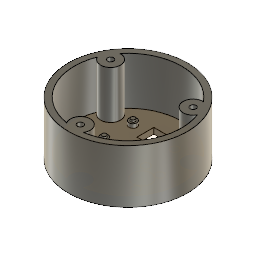
Module (Autodesk Fusion 360 design; units mm, degrees)
Autodesk Fusion 360 part; units mm, degrees
note: some values were not read from the file. Set by a fixed rule: which sketch regions a step uses.
sketch "Sketch1" plane through (0, 0, 0) normal (0, 0, 1) x (1, 0, 0)
  circle A0 centre (0, 0) radius 30
  dimension "d1" = 60
  measures "d1" diameter of A0
extrude "Extrude1" add sketch "Sketch1" along normal blind 27
sketch "Sketch2" plane through (0, 0, 0) normal (0, 0, -1) x (1, 0, 0)
  circle A0 centre (0, 0) radius 30
  line L0 (0, 24) -> (-20.7846, 12)
  line L1 (-20.7846, 12) -> (-20.7846, -12)
  line L2 (-20.7846, -12) -> (0, -24)
  line L3 (0, -24) -> (20.7846, -12)
  line L4 (20.7846, -12) -> (20.7846, 12)
  line L5 (20.7846, 12) -> (0, 24)
  circle A1 centre (0, 24) radius 1.5
  circle A2 centre (20.7846, -12) radius 1.5
  circle A3 centre (-20.7846, -12) radius 1.5
  dimension "d4" = 3
  dimension "d5" = 3
  dimension "d6" = 3
  measures "d4" diameter of A1
  measures "d5" diameter of A2
  measures "d6" diameter of A3
extrude "Extrude2" cut sketch "Sketch2" against normal blind 30 contours L0 L5 A1 | L0 L5 A1 | L1 L2 A3 | L1 L2 A3 | L3 L4 A2 | L3 L4 A2
sketch "Sketch3" plane through (0, 0, 0) normal (0, 0, -1) x (1, 0, 0)
  circle A0 centre (0, 24) radius 1.5
  circle A1 centre (20.7846, -12) radius 1.5
  circle A2 centre (-20.7846, -12) radius 1.5
  circle A3 centre (0, 0) radius 30
  line L0 (2.25, 25.299) -> (0, 26.5981)
  line L1 (0, 26.5981) -> (-2.25, 25.299)
  line L2 (-2.25, 25.299) -> (-2.25, 22.701)
  line L3 (-2.25, 22.701) -> (0, 21.4019)
  line L4 (0, 21.4019) -> (2.25, 22.701)
  line L5 (2.25, 22.701) -> (2.25, 25.299)
  line L6 (23.0821, -10.7869) -> (20.8828, -9.4038)
  line L7 (20.8828, -9.4038) -> (18.5853, -10.6169)
  line L8 (18.5853, -10.6169) -> (18.4871, -13.2131)
  line L9 (18.4871, -13.2131) -> (20.6864, -14.5962)
  line L10 (20.6864, -14.5962) -> (22.9839, -13.3831)
  line L11 (22.9839, -13.3831) -> (23.0821, -10.7869)
  line L12 (-18.5346, -10.701) -> (-20.7846, -9.4019)
  line L13 (-20.7846, -9.4019) -> (-23.0346, -10.701)
  line L14 (-23.0346, -10.701) -> (-23.0346, -13.299)
  line L15 (-23.0346, -13.299) -> (-20.7846, -14.5981)
  line L16 (-20.7846, -14.5981) -> (-18.5346, -13.299)
  line L17 (-18.5346, -13.299) -> (-18.5346, -10.701)
  dimension "d9" = 2.25
  dimension "d10" = 2.25
  dimension "d11" = 2.25
  measures "d9" distance of A3.centre L5
  measures "d10" distance of L11
  measures "d11" distance of L17
extrude "Extrude3" cut sketch "Sketch3" against normal blind 2.4 contours L0 L1 L2 L3 L4 L5 | L6 L7 L8 L9 L10 L11 | L12 L13 L14 L15 L16 L17
sketch "Sketch5" plane through (0, 0, 27) normal (0, 0, 1) x (-1, 0, 0)
  circle A0 centre (0, 24) radius 1.5
  circle A1 centre (-20.7846, -12) radius 1.5
  circle A2 centre (20.7846, -12) radius 1.5
  circle A3 centre (0, 0) radius 30
  circle A4 centre (0, 0) radius 27
  circle A5 centre (0, 24) radius 5
  circle A6 centre (-20.7846, -12) radius 5
  circle A7 centre (20.7846, -12) radius 5
  dimension "d14" = 10
  dimension "d15" = 10
  dimension "d16" = 10
  measures "d14" diameter of A5
  measures "d15" diameter of A6
  measures "d16" diameter of A7
extrude "Extrude4" cut sketch "Sketch5" against normal blind 24 contours A4 A5 A6 A7
sketch "Sketch7" plane through (0, 0, 3) normal (0, 0, 1) x (-1, 0, 0)
  arc A0 (-4.2295, 26.6667) -> (-25.2088, -9.6705) centre (0, 0) ccw
  arc A1 (-20.9792, -16.9962) -> (-25.2088, -9.6705) centre (-20.7846, -12) ccw
  arc A2 (-20.9792, -16.9962) -> (20.9792, -16.9962) centre (0, 0) ccw
  arc A3 (25.2088, -9.6705) -> (20.9792, -16.9962) centre (20.7846, -12) ccw
  arc A4 (25.2088, -9.6705) -> (4.2295, 26.6667) centre (0, 0) ccw
  arc A5 (-4.2295, 26.6667) -> (4.2295, 26.6667) centre (0, 24) ccw
  line L0 (-4.25, -8.75) -> (4.25, -8.75)
  line L1 (4.25, -8.75) -> (4.25, -17.25)
  line L2 (4.25, -17.25) -> (-4.25, -17.25)
  line L3 (-4.25, -17.25) -> (-4.25, -8.75)
  line L4 (-4.25, -8.75) -> (4.25, -17.25) construction
  line L5 (4.25, -8.75) -> (-4.25, -17.25) construction
  dimension "d22" = 8.5
  dimension "d23" = 8.5
extrude "Extrude5" cut sketch "Sketch7" against normal blind 5 contours L0 L1 L2 L3
sketch "Sketch8" plane through (0, 0, 3) normal (0, 0, 1) x (-1, 0, 0)
  line L0 (4.25, -8.75) -> (4.25, -17.25)
  line L1 (4.25, -17.25) -> (-4.25, -17.25)
  line L2 (-4.25, -17.25) -> (-4.25, -8.75)
  line L3 (-4.25, -8.75) -> (4.25, -8.75)
  arc A0 (-4.2295, 26.6667) -> (-25.2088, -9.6705) centre (0, 0) ccw
  arc A1 (-20.9792, -16.9962) -> (-25.2088, -9.6705) centre (-20.7846, -12) ccw
  arc A2 (-20.9792, -16.9962) -> (20.9792, -16.9962) centre (0, 0) ccw
  arc A3 (25.2088, -9.6705) -> (20.9792, -16.9962) centre (20.7846, -12) ccw
  arc A4 (25.2088, -9.6705) -> (4.2295, 26.6667) centre (0, 0) ccw
  arc A5 (-4.2295, 26.6667) -> (4.2295, 26.6667) centre (0, 24) ccw
  line L4 (5, -5) -> (8, -5)
  line L5 (8, -5) -> (8, -21)
  line L6 (8, -21) -> (5, -21)
  line L7 (5, -21) -> (5, -5)
  line L8 (5, -21) -> (-5, -21)
  line L9 (-5, -21) -> (-5, -18)
  line L10 (-5, -18) -> (5, -18)
  line L11 (5, -18) -> (5, -21)
  line L12 (-5, -21) -> (-8, -21)
  line L13 (-8, -21) -> (-8, -5)
  line L14 (-8, -5) -> (-5, -5)
  line L15 (-5, -5) -> (-5, -21)
sketch "Sketch9" plane through (0, 0, 3) normal (0, 0, 1) x (-1, 0, 0)
  line L0 (4.25, -8.75) -> (4.25, -17.25)
  line L1 (4.25, -17.25) -> (-4.25, -17.25)
  line L2 (-4.25, -17.25) -> (-4.25, -8.75)
  line L3 (-4.25, -8.75) -> (4.25, -8.75)
  arc A0 (-4.2295, 26.6667) -> (-25.2088, -9.6705) centre (0, 0) ccw
  arc A1 (-20.9792, -16.9962) -> (-25.2088, -9.6705) centre (-20.7846, -12) ccw
  arc A2 (-20.9792, -16.9962) -> (20.9792, -16.9962) centre (0, 0) ccw
  arc A3 (25.2088, -9.6705) -> (20.9792, -16.9962) centre (20.7846, -12) ccw
  arc A4 (25.2088, -9.6705) -> (4.2295, 26.6667) centre (0, 0) ccw
  arc A5 (-4.2295, 26.6667) -> (4.2295, 26.6667) centre (0, 24) ccw
  circle A6 centre (-15, 8) radius 4.7
  dimension "d28" = 9.4
  measures "d28" diameter of A6
extrude "Extrude7" cut sketch "Sketch9" against normal blind 5 contours A6
sketch "Sketch10" plane through (0, 0, 3) normal (0, 0, 1) x (-1, 0, 0)
  circle A0 centre (-15, 8) radius 4.7
  line L0 (4.25, -8.75) -> (4.25, -17.25)
  line L1 (4.25, -17.25) -> (-4.25, -17.25)
  line L2 (-4.25, -17.25) -> (-4.25, -8.75)
  line L3 (-4.25, -8.75) -> (4.25, -8.75)
  arc A1 (-4.2295, 26.6667) -> (-25.2088, -9.6705) centre (0, 0) ccw
  arc A2 (-20.9792, -16.9962) -> (-25.2088, -9.6705) centre (-20.7846, -12) ccw
  arc A3 (-20.9792, -16.9962) -> (20.9792, -16.9962) centre (0, 0) ccw
  arc A4 (25.2088, -9.6705) -> (20.9792, -16.9962) centre (20.7846, -12) ccw
  arc A5 (25.2088, -9.6705) -> (4.2295, 26.6667) centre (0, 0) ccw
  arc A6 (-4.2295, 26.6667) -> (4.2295, 26.6667) centre (0, 24) ccw
  circle A7 centre (-18, 14) radius 2
  circle A8 centre (-18, 2) radius 2
  dimension "d31" = 4
  dimension "d32" = 4
  measures "d31" diameter of A7
  measures "d32" diameter of A8
extrude "Extrude8" add sketch "Sketch10" along normal blind 11.5 contours A7 | A8
sketch "Sketch13" plane through (0, 0, 3) normal (0, 0, 1) x (-1, 0, 0)
  circle A0 centre (-18, 14) radius 2
  circle A1 centre (-18, 2) radius 2
  circle A2 centre (-15, 8) radius 4.7
  line L0 (4.25, -8.75) -> (4.25, -17.25)
  line L1 (4.25, -17.25) -> (-4.25, -17.25)
  line L2 (-4.25, -17.25) -> (-4.25, -8.75)
  line L3 (-4.25, -8.75) -> (4.25, -8.75)
  arc A3 (-4.2295, 26.6667) -> (-25.2088, -9.6705) centre (0, 0) ccw
  arc A4 (-20.9792, -16.9962) -> (-25.2088, -9.6705) centre (-20.7846, -12) ccw
  arc A5 (-20.9792, -16.9962) -> (20.9792, -16.9962) centre (0, 0) ccw
  arc A6 (25.2088, -9.6705) -> (20.9792, -16.9962) centre (20.7846, -12) ccw
  arc A7 (25.2088, -9.6705) -> (4.2295, 26.6667) centre (0, 0) ccw
  arc A8 (-4.2295, 26.6667) -> (4.2295, 26.6667) centre (0, 24) ccw
  line L4 (0, -13) -> (-10.5, -13)
  line L5 (-10.5, -13) -> (-10.5, 1.5)
  line L6 (-10.5, 1.5) -> (0, 1.5)
  line L7 (0, 1.5) -> (0, -13)
  line L8 (0, -13) -> (10.5, -13)
  line L9 (10.5, -13) -> (10.5, 1.5)
  line L10 (10.5, 1.5) -> (0, 1.5)
  line L11 (0, 1.5) -> (0, -13)
  circle A9 centre (10.5, 1.5) radius 2
  circle A10 centre (-10.5, 1.5) radius 2
  circle A11 centre (10.5, -13) radius 2
  circle A12 centre (-10.5, -13) radius 2
  dimension "d35" = 14.5
  dimension "d36" = 10.5
  dimension "d37" = 14.5
  dimension "d38" = 4
  dimension "d39" = 4
  dimension "d40" = 4
  dimension "d41" = 4
  measures "d38" diameter of A9
  measures "d39" diameter of A10
  measures "d40" diameter of A11
  measures "d41" diameter of A12
extrude "Extrude9" add sketch "Sketch13" along normal blind 2 contours L8 L9 A11 | L8 L9 A11 | L5 L6 A10 | L5 L6 A10 | L9 L10 A9 | L9 L10 A9 | L4 L5 A12 | L4 L5 A12
sketch "Sketch14" plane through (0, 0, 5) normal (0, 0, 1) x (-1, 0, 0)
  circle A0 centre (10.5, -13) radius 2
  circle A1 centre (10.5, -13) radius 1.1
  circle A2 centre (-10.5, -13) radius 1.1
  circle A3 centre (10.5, 1.5) radius 1.1
  circle A4 centre (-10.5, 1.5) radius 1.1
  dimension "d44" = 2.2
  dimension "d45" = 2.2
  dimension "d46" = 2.2
  dimension "d47" = 2.2
  measures "d44" diameter of A1
  measures "d45" diameter of A2
  measures "d46" diameter of A3
  measures "d47" diameter of A4
extrude "Extrude10" add sketch "Sketch14" along normal blind 1 contours A1 | A2 | A3 | A4
sketch "Sketch15" plane through (0, 0, 14.5) normal (0, 0, 1) x (-1, 0, 0)
  circle A0 centre (-18, 2) radius 2
  circle A1 centre (-18, 2) radius 1.1
  circle A2 centre (-18, 14) radius 1.1
  dimension "d50" = 2.2
  dimension "d51" = 2.2
  measures "d50" diameter of A1
  measures "d51" diameter of A2
extrude "Extrude11" add sketch "Sketch15" along normal blind 1 contours A1 | A2
sketch "Sketch16" plane through (0, 0, 3) normal (0, 0, 1) x (-1, 0, 0)
  circle A0 centre (-10.5, -13) radius 2
  circle A1 centre (10.5, -13) radius 2
  circle A2 centre (-10.5, 1.5) radius 2
  circle A3 centre (10.5, 1.5) radius 2
  circle A4 centre (-18, 14) radius 2
  circle A5 centre (-18, 2) radius 2
  circle A6 centre (-15, 8) radius 4.7
  line L0 (4.25, -8.75) -> (4.25, -17.25)
  line L1 (4.25, -17.25) -> (-4.25, -17.25)
  line L2 (-4.25, -17.25) -> (-4.25, -8.75)
  line L3 (-4.25, -8.75) -> (4.25, -8.75)
  arc A7 (-4.2295, 26.6667) -> (-25.2088, -9.6705) centre (0, 0) ccw
  arc A8 (-20.9792, -16.9962) -> (-25.2088, -9.6705) centre (-20.7846, -12) ccw
  arc A9 (-20.9792, -16.9962) -> (20.9792, -16.9962) centre (0, 0) ccw
  arc A10 (25.2088, -9.6705) -> (20.9792, -16.9962) centre (20.7846, -12) ccw
  arc A11 (25.2088, -9.6705) -> (4.2295, 26.6667) centre (0, 0) ccw
  arc A12 (-4.2295, 26.6667) -> (4.2295, 26.6667) centre (0, 24) ccw
sketch "Sketch12" plane through (0, 0, 3) normal (0, 0, 1) x (-1, 0, 0)
  circle A0 centre (-18, 11) radius 2
  circle A1 centre (-18, -1) radius 2
  circle A2 centre (-15, 5) radius 4.7
  line L0 (4.25, -8.75) -> (4.25, -17.25)
  line L1 (4.25, -17.25) -> (-4.25, -17.25)
  line L2 (-4.25, -17.25) -> (-4.25, -8.75)
  line L3 (-4.25, -8.75) -> (4.25, -8.75)
  arc A3 (-4.2295, 26.6667) -> (-25.2088, -9.6705) centre (0, 0) ccw
  arc A4 (-20.9792, -16.9962) -> (-25.2088, -9.6705) centre (-20.7846, -12) ccw
  arc A5 (-20.9792, -16.9962) -> (20.9792, -16.9962) centre (0, 0) ccw
  arc A6 (25.2088, -9.6705) -> (20.9792, -16.9962) centre (20.7846, -12) ccw
  arc A7 (25.2088, -9.6705) -> (4.2295, 26.6667) centre (0, 0) ccw
  arc A8 (-4.2295, 26.6667) -> (4.2295, 26.6667) centre (0, 24) ccw
sketch "Sketch6" plane through (0, 0, 3) normal (0, 0, 1) x (-1, 0, 0)
  arc A0 (-4.2295, 26.6667) -> (-25.2088, -9.6705) centre (0, 0) ccw
  arc A1 (-20.9792, -16.9962) -> (-25.2088, -9.6705) centre (-20.7846, -12) ccw
  arc A2 (-20.9792, -16.9962) -> (20.9792, -16.9962) centre (0, 0) ccw
  arc A3 (25.2088, -9.6705) -> (20.9792, -16.9962) centre (20.7846, -12) ccw
  arc A4 (25.2088, -9.6705) -> (4.2295, 26.6667) centre (0, 0) ccw
  arc A5 (-4.2295, 26.6667) -> (4.2295, 26.6667) centre (0, 24) ccw
  line L0 (0, -17) -> (14.7224, -8.5)
  line L1 (14.7224, -8.5) -> (14.7224, 8.5)
  line L2 (14.7224, 8.5) -> (0, 17)
  line L3 (0, 17) -> (-14.7224, 8.5)
  line L4 (-14.7224, 8.5) -> (-14.7224, -8.5)
  line L5 (-14.7224, -8.5) -> (0, -17)
  line L6 (4.25, -21.25) -> (4.25, -12.75)
  line L7 (-4.25, -21.25) -> (4.25, -12.75) construction
  line L8 (4.25, -21.25) -> (-4.25, -12.75) construction
  circle A6 centre (-14.7224, 8.5) radius 4.7
  dimension "d19" = 8.5
  dimension "d20" = 8.5
  dimension "d21" = 9.4
  measures "d21" diameter of A6
sketch "Sketch4" plane through (0, 0, 0) normal (0, 0, -1) x (1, 0, 0)
  line L0 (-20.7846, -9.4019) -> (-18.5346, -10.701)
  line L1 (-18.5346, -10.701) -> (-18.5346, -13.299)
  line L2 (-18.5346, -13.299) -> (-20.7846, -14.5981)
  line L3 (-20.7846, -14.5981) -> (-23.0346, -13.299)
  line L4 (-23.0346, -13.299) -> (-23.0346, -10.701)
  line L5 (-23.0346, -10.701) -> (-20.7846, -9.4019)
  line L6 (0, 26.5981) -> (2.25, 25.299)
  line L7 (2.25, 25.299) -> (2.25, 22.701)
  line L8 (2.25, 22.701) -> (0, 21.4019)
  line L9 (0, 21.4019) -> (-2.25, 22.701)
  line L10 (-2.25, 22.701) -> (-2.25, 25.299)
  line L11 (-2.25, 25.299) -> (0, 26.5981)
  line L12 (20.8828, -9.4038) -> (23.0821, -10.7869)
  line L13 (23.0821, -10.7869) -> (22.9839, -13.3831)
  line L14 (22.9839, -13.3831) -> (20.6864, -14.5962)
  line L15 (20.6864, -14.5962) -> (18.4871, -13.2131)
  line L16 (18.4871, -13.2131) -> (18.5853, -10.6169)
  line L17 (18.5853, -10.6169) -> (20.8828, -9.4038)
  circle A0 centre (0, 0) radius 30
